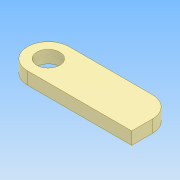
# Autodesk Inventor part: Selection_Lever 2
Saved by Autodesk Inventor 2018.1 (Build 221171000, 171)
## iProperties
Created: 2019-02-14
Part Number: Selection_Lever 2
Material: Nylon 6/6
Document SubType Name: Modeling
Designer: James
Density: 1.13 g/cm^3
Appearance: Nylon 6
Mass: 0.938475 g
Surface Area: 8.02633 cm^2
Volume: 0.830509 cm^3
Author: James
Autodesk Inventor part; units mm, degrees
ref_plane "YZ Plane" through (0, 0, 0) normal (1, 0, 0) x (0, 1, 0)
ref_plane "XZ Plane" through (0, 0, 0) normal (0, 1, 0) x (-1, 0, 0)
ref_plane "XY Plane" through (0, 0, 0) normal (0, 0, 1) x (1, 0, 0)
sketch "Sketch1" plane through (0, 0, 0) normal (0, 0, 1) x (1, 0, 0)
  line L0 (0, 0) -> (30, 0)
  line L1 (30, 0) -> (30, 10)
  line L2 (30, 10) -> (0, 10)
  line L3 (0, 10) -> (0, 0)
  dimension "d0" = 30
  dimension "d1" = 10
  constraints: 8 end point, 2 parallel, 1 horizontal, 1 perpendicular
  measures "d0" distance of L1.end L2.end
  measures "d1" distance of L0.end L1.end
extrude "Extrusion1" add sketch "Sketch1" along normal blind 3
sketch "Sketch2" plane through (0, 0, 3) normal (0, 0, 1) x (1, 0, 0)
  line L0 (30, 10) -> (0, 10) projected
  line L1 (0, 0) -> (30, 0) projected
  line L2 (0, 10) -> (0, 0) projected
  point P0 (5, 5)
  dimension "d4" = 5
  dimension "d5" = 5
  dimension "d6" = 5
  measures "d4" distance from line of point (5, 5) L0
  measures "d5" distance from line of L1 point (5, 5)
  measures "d6" distance from line of L2 point (5, 5)
hole "Hole1" at (5, 5, 3) direction (0, 0, -1) diameter 5.5 end through all
full round fillet "Fillet1" first side at (20, 10, 1) centre faces at (0, 6.6667, 1) second side at (10, 0, 2)
fillet "Fillet2" radius 5 1 edges at (30, 10, 1.5)
equation "\"d4\" = d5"
body "Solid1"
